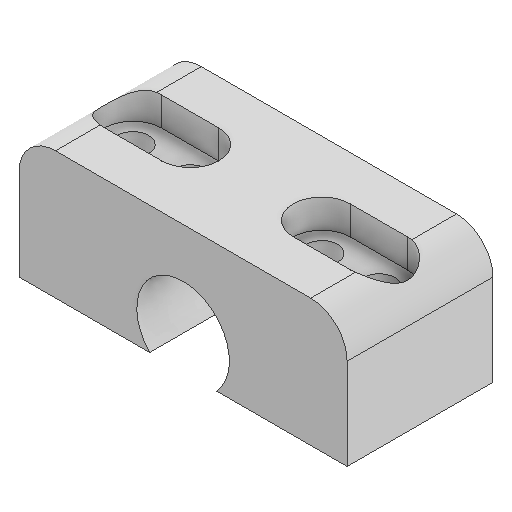
# Autodesk Inventor part: hoverboardMotorMount
Saved by Autodesk Inventor 2025 (Build 290162000, 162)
## iProperties
Created: 2024-10-15
Part Number: hoverboardMotorMount
Material: Generic
Document SubType Name: Modeling
Designer: derm
Density: 1 g/cm^3
Appearance: Default
Author: derm
Autodesk Inventor part; units mm, degrees
ref_plane "YZ Plane" through (0, 0, 0) normal (1, 0, 0) x (0, 1, 0)
ref_plane "XZ Plane" through (0, 0, 0) normal (0, 1, 0) x (-1, 0, 0)
ref_plane "XY Plane" through (0, 0, 0) normal (0, 0, 1) x (1, 0, 0)
sketch "Sketch1" plane through (0, 0, 0) normal (0, 0, 1) x (1, 0, 0)
  arc A0 (5.8166, -5.586) -> (-5.8166, -5.586) centre (0, 0) ccw
  line L0 (-5.8166, -5.586) -> (5.8166, -5.586)
  line L1 (0, -5.586) -> (-28.575, -5.586)
  line L2 (-28.575, -5.586) -> (-28.575, 16.639)
  line L3 (-28.575, 16.639) -> (0, 16.639)
  line L4 (0, 16.639) -> (0, -5.586)
  line L5 (0, -5.586) -> (28.575, -5.586)
  line L6 (28.575, -5.586) -> (28.575, 16.639)
  line L7 (28.575, 16.639) -> (0, 16.639)
  line L8 (0, 16.639) -> (0, -5.586)
  point P0 (-5.8166, -5.586)
  dimension "d0" = 16.129
  dimension "d1" = 11.6332
  dimension "d2" = 57.15
  dimension "d3" = 22.225
  dimension "d4" = 22.225
  constraints: 18 end point, 4 parallel, 3 horizontal, 2 perpendicular, 2 point on circle, 1 centre point, 1 coincident, 1 collinear, 1 midpoint
  measures "d0" diameter of A0
  measures "d1" distance of L0.start L0.end
  measures "d2" distance between parallel lines of L6 L2
  measures "d3" distance between parallel lines of L1 L3
  measures "d4" distance of L5.end L6.end
extrude "Extrusion1" add sketch "Sketch1" against normal blind 25.4 contours A0 L4 L7 L6 L5 | A0 L1 L2 L3 L4
sketch "Sketch2" plane through (5.8166, -5.586, 0) normal (0, -1, 0) x (1, 0, 0)
  line L0 (-13.8811, 0) -> (2.2479, 0) projected
  line L1 (0, 0) -> (22.7584, 0) projected
  line L2 (0, 0) -> (0, -25.4) projected
  line L3 (22.7584, -25.4) -> (0, -25.4) projected
  line L4 (22.7584, 0) -> (22.7584, -25.4) projected
  line L5 (-34.3916, 0) -> (-11.6332, 0) projected
  line L6 (-34.3916, 0) -> (-34.3916, -25.4) projected
  line L7 (-11.6332, -25.4) -> (-34.3916, -25.4) projected
  line L8 (-11.6332, 0) -> (-11.6332, -25.4) projected
  circle A0 centre (15.6282, -12.7) radius 2.75
  circle A1 centre (5.6282, -12.7) radius 2.75
  point P0 (-5.8166, 0)
  dimension "d7" = 5.5
  dimension "d8" = 5.5
  dimension "d9" = 10
  constraints: 2 centre point
  measures "d7" diameter of A1
  measures "d8" diameter of A0
  measures "d9" distance of A0.centre A1.centre
extrude "Extrusion2" cut sketch "Sketch2" along normal through all both and the other way through all contours A0 | A1
ref_plane "Work Plane1" through (0, -5.586, 0) normal (1, 0, 0) x (0, 0, -1)
sketch "Sketch3" plane through (-28.575, 16.639, 0) normal (0, 1, 0) x (1, 0, 0)
  circle A0 centre (40.0198, 12.7) radius 2.75 projected
  circle A1 centre (50.0198, 12.7) radius 2.75 projected
  line L0 (57.15, 0) -> (0, 0) projected
  line L1 (57.15, 0) -> (57.15, 25.4) projected
  line L2 (0, 25.4) -> (57.15, 25.4) projected
  line L3 (0, 0) -> (0, 25.4) projected
  line L4 (40.0198, 12.7) -> (50.0198, 12.7) construction
  line L5 (40.0198, 7.7307) -> (50.0198, 7.7307)
  line L6 (50.0198, 17.6693) -> (40.0198, 17.6693)
  arc A2 (40.0198, 17.6693) -> (40.0198, 7.7307) centre (40.0198, 12.7) ccw
  arc A3 (50.0198, 7.7307) -> (50.0198, 17.6693) centre (50.0198, 12.7) ccw
  point P0 (28.575, 0)
  point P1 (45.0198, 12.7)
  constraints: 8 end point, 4 point on circle, 4 tangent, 2 centre point, 1 horizontal, 1 midpoint, 1 parallel
extrude "Extrusion3" cut sketch "Sketch3" against normal blind 5 contours A2 L6 A3 L5
mirror "Mirror1" about plane through (0, -5.586, 0) normal (1, 0, 0) of "Extrusion2", "Extrusion3"
fillet "Fillet1" radius 6.35 2 edges at (-28.575, 16.639, -12.7) (28.575, 16.639, -12.7)
body "Solid1"
